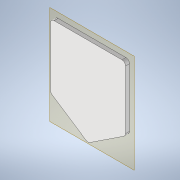
# Autodesk Inventor part: Cover_Robot_Motor_Shoulder
Saved by Autodesk Inventor 2022.2 (Build 262287010, 287A)
## iProperties
Created: 2024-07-23
Part Number: Cover_Robot_Motor_Shoulder
Material: Generisch
Document SubType Name: Modeling
Designer: ppovolni
Density: 1 g/cm^3
Appearance: Vorgabe
Author: ppovolni
Autodesk Inventor part; units mm, degrees
ref_plane "YZ Plane" through (0, 0, 0) normal (1, 0, 0) x (0, 1, 0)
ref_plane "XZ Plane" through (0, 0, 0) normal (0, 1, 0) x (-1, 0, 0)
ref_plane "XY Plane" through (0, 0, 0) normal (0, 0, 1) x (1, 0, 0)
ref_plane "Arbeitsebene1" through (0, 0, 0) normal (0, 0, 1) x (1, 0, 0)
sketch "Skizze1" plane through (0, 0, 0) normal (0, 0, 1) x (1, 0, 0)
  line L0 (9.1071, 105.908) -> (0.6071, 100.2819) construction
  arc A0 (9.1071, 105.908) -> (9.6, 106.8252) centre (8.5, 106.8252) ccw construction
  line L1 (9.6, 121.5) -> (9.6, 106.8252) construction
  arc A1 (9.6, 121.5) -> (8.5, 122.6) centre (8.5, 121.5) ccw construction
  line L2 (-8.5, 122.6) -> (8.5, 122.6) construction
  arc A2 (-8.5, 122.6) -> (-9.6, 121.5) centre (-8.5, 121.5) ccw construction
  line L3 (-9.6, 106.8252) -> (-9.6, 121.5) construction
  arc A3 (-9.6, 106.8252) -> (-9.1071, 105.908) centre (-8.5, 106.8252) ccw construction
  line L4 (-0.6071, 100.2819) -> (-9.1071, 105.908) construction
  arc A4 (-0.6071, 100.2819) -> (0.6071, 100.2819) centre (0, 101.1992) ccw construction
  circle A5 centre (5.6569, 118.6569) radius 1.6 construction
  circle A6 centre (5.6569, 107.3431) radius 1.6 construction
  circle A7 centre (-5.6569, 107.3431) radius 1.6 construction
  circle A8 centre (-5.6569, 118.6569) radius 1.6 construction
  circle A9 centre (0, 113) radius 3 construction
  arc A10 (-8.5, 122.4) -> (-9.4, 121.5) centre (-8.5, 121.5) ccw
  line L5 (-8.5, 122.4) -> (8.5, 122.4)
  arc A11 (9.4, 121.5) -> (8.5, 122.4) centre (8.5, 121.5) ccw
  line L6 (9.4, 121.5) -> (9.4, 106.8252)
  arc A12 (8.9967, 106.0747) -> (9.4, 106.8252) centre (8.5, 106.8252) ccw
  line L7 (8.9967, 106.0747) -> (0.4967, 100.4487)
  arc A13 (-0.4967, 100.4487) -> (0.4967, 100.4487) centre (0, 101.1992) ccw
  line L8 (-0.4967, 100.4487) -> (-8.9967, 106.0747)
  arc A14 (-9.4, 106.8252) -> (-8.9967, 106.0747) centre (-8.5, 106.8252) ccw
  line L9 (-9.4, 106.8252) -> (-9.4, 121.5)
  point P0 (0, 0)
  dimension "d2" = 0
  dimension "d0" = 0.2
  constraints: 10 end point, 10 point on circle, 5 centre point, 9 other
  measures "d0" distance between parallel lines of L3 L9
extrude "Extrusion1" add sketch "Skizze1" along normal blind 1
